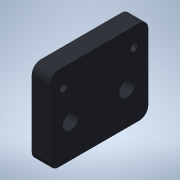
# Autodesk Inventor part: Standard
Saved by Autodesk Inventor 2020.3 (Build 243373000, 373)
## iProperties
RuleStatus: InUse
AfterDocSave0: file://Part Number Cleaner
Created: 2022-02-02
Material: ABS, BLACK
Catalog Web Link: https://www.janelia.org/
Vendor: HHMI: JRC - jET
Document SubType Name: Modeling
Designer: solomone
Density: 1.06 g/cm^3
Appearance: Black Anodize
LAB/DEPT: A. LEE (LAB)
DESIGN DEPARTMENT: HHMI: JRC - jET
ALTERED ITEM PART NUMBER: N/A
ALTERED ITEM VENDOR: N/A
ALTERED ITEM DESCRIPTION: N/A
Title: Standard
Author: solomone
Revision Number: 0
Autodesk Inventor part; units mm, degrees
ref_plane "YZ Plane" through (0, 0, 0) normal (1, 0, 0) x (0, 1, 0)
ref_plane "XZ Plane" through (0, 0, 0) normal (0, 1, 0) x (-1, 0, 0)
ref_plane "XY Plane" through (0, 0, 0) normal (0, 0, 1) x (1, 0, 0)
sketch "Sketch1" plane through (0, 0, 0) normal (1, 0, 0) x (0, 1, 0)
  line L0 (-12, 17.5) -> (18, 17.5)
  line L1 (18, 17.5) -> (18, -17.5)
  line L2 (18, -17.5) -> (-12, -17.5)
  line L3 (-12, -17.5) -> (-12, 17.5)
  point P0 (0, 0)
  dimension "d0" = 35
  dimension "d1" = 30
  dimension "d3" = 17.5
  dimension "d7" = 18
  constraints: 8 end point, 2 parallel, 1 horizontal, 1 perpendicular
  measures "d0" distance of L2.end L0.start
  measures "d1" distance of L0.start L0.end
  measures "d3" distance from line of point (0, 0) L0
  measures "d7" distance from line of L1 point (0, 0)
extrude "Extrusion1" add sketch "Sketch1" along normal blind 6.35
fillet "Fillet1" radius 3.175 4 edges at (3.175, -12, -17.5) (3.175, -12, 17.5) (3.175, 18, 17.5) (3.175, 18, -17.5)
sketch "Sketch2" plane through (6.35, 0, 0) normal (1, 0, 0) x (0, 0, -1)
  point P0 (0, 0)
  point P1 (-10, 0)
  point P2 (10, 0)
  dimension "d15" = 20
  dimension "d16" = 10
  constraints: 2 horizontal alignment
  measures "d15" distance of point (10, 0) point (-10, 0)
  measures "d16" distance of point (10, 0) point (0, 0)
hole "Hole1" at (6.35, 0, 10) at (6.35, 0, -10) direction (-1, 0, 0) diameter 5.5118 end through all clearance for "Hex Head Bolt" size "M5" standard "Ansi Metric M Profile"
sketch "Sketch3" plane through (6.35, 0, 0) normal (1, 0, 0) x (0, 0, -1)
  point P0 (0, 0)
  point P1 (-12.5, 11.43)
  point P2 (12.5, 11.43)
  dimension "d17" = 25
  dimension "d18" = 12.5
  dimension "d19" = 11.43
  constraints: 1 horizontal alignment
  measures "d17" distance of point (12.5, 11.43) point (-12.5, 11.43)
  measures "d18" horizontal distance of point (0, 0) point (-12.5, 11.43)
  measures "d19" vertical distance of point (0, 0) point (-12.5, 11.43)
hole "Hole2" at (6.35, 11.43, 12.5) at (6.35, 11.43, -12.5) direction (-1, 0, 0) diameter 2.459 end through all thread size "M3x0.5" class "6H" standard "ANSI Metric M Profile"
equation "\"d3\" = 0.5 * d0"
equation "\"d16\" = 0.5 * d15"
equation "\"d18\" = 0.5 * d17"
body "Solid1"
